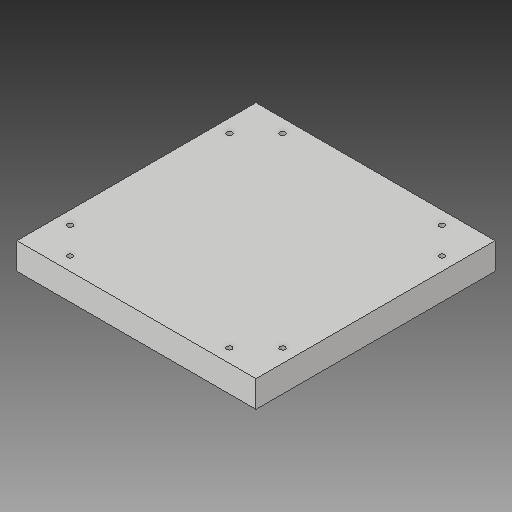
# Autodesk Inventor part: 内层升降板
Saved by Autodesk Inventor 2017 (Build 210142000, 142)
## iProperties
Part Number: 内层升降板
Material: 常规
Document SubType Name: Modeling
Designer: PANDA
Density: 1 g/cm^3
Appearance: 默认
Mass: 645.989 g
Surface Area: 810.096 cm^2
Volume: 645.989 cm^3
Author: PANDA
Autodesk Inventor part; units mm, degrees
ref_plane "YZ Plane" through (0, 0, 0) normal (1, 0, 0) x (0, 1, 0)
ref_plane "XZ Plane" through (0, 0, 0) normal (0, 1, 0) x (-1, 0, 0)
ref_plane "XY Plane" through (0, 0, 0) normal (0, 0, 1) x (1, 0, 0)
sketch "草图2" plane through (0, 0, 0) normal (0, 1, 0) x (-1, 0, 0)
  line L0 (90, 90) -> (-90, 90)
  line L1 (-90, 90) -> (-90, -90)
  line L2 (-90, -90) -> (90, -90)
  line L3 (90, -90) -> (90, 90)
  point P0 (0, 0)
  dimension "d4" = 180
  dimension "d5" = 180
  constraints: 8 end point, 2 parallel, 1 horizontal, 1 perpendicular
  measures "d4" distance of L2.end L1.end
  measures "d5" distance of L1.end L0.end
extrude "拉伸2" add sketch "草图2" along normal blind 20
sketch "草图3" plane through (0, 20, 0) normal (0, 1, 0) x (1, 0, 0)
  circle A0 centre (80, 60) radius 2
  point P0 (0, 0)
  dimension "d8" = 4
  constraints: 1 centre point
  measures "d8" diameter of A0
extrude "拉伸3" cut sketch "草图3" against normal through all
sketch "草图4" plane through (0, 0, 0) normal (0, -1, 0) x (1, 0, 0)
  circle A0 centre (60, -80) radius 2
  point P0 (0, 0)
  dimension "d11" = 4
  constraints: 1 centre point
  measures "d11" diameter of A0
extrude "拉伸4" cut sketch "草图4" against normal through all
sketch "草图5" plane through (0, 0, 0) normal (0, -1, 0) x (1, 0, 0)
  circle A0 centre (80, 60) radius 2
  point P0 (0, 0)
  dimension "d14" = 4
  constraints: 1 centre point
  measures "d14" diameter of A0
extrude "拉伸5" cut sketch "草图5" against normal through all
sketch "草图6" plane through (0, 0, 0) normal (0, -1, 0) x (1, 0, 0)
  circle A0 centre (60, 80) radius 2
  point P0 (0, 0)
  dimension "d17" = 4
  constraints: 1 centre point
  measures "d17" diameter of A0
extrude "拉伸6" cut sketch "草图6" against normal through all
sketch "草图7" plane through (0, 0, 0) normal (0, -1, 0) x (1, 0, 0)
  circle A0 centre (-80, -60) radius 2
  point P0 (0, 0)
  dimension "d20" = 4
  constraints: 1 centre point
  measures "d20" diameter of A0
extrude "拉伸7" cut sketch "草图7" against normal through all
sketch "草图8" plane through (0, 0, 0) normal (0, -1, 0) x (1, 0, 0)
  circle A0 centre (-60, -80) radius 2
  point P0 (0, 0)
  dimension "d23" = 4
  constraints: 1 centre point
  measures "d23" diameter of A0
extrude "拉伸8" cut sketch "草图8" against normal through all
sketch "草图9" plane through (0, 0, 0) normal (0, -1, 0) x (1, 0, 0)
  circle A0 centre (-80, 60) radius 2
  point P0 (0, 0)
  dimension "d26" = 4
  constraints: 1 centre point
  measures "d26" diameter of A0
extrude "拉伸9" cut sketch "草图9" against normal through all
sketch "草图10" plane through (0, 0, 0) normal (0, -1, 0) x (1, 0, 0)
  circle A0 centre (-60, 80) radius 2
  point P0 (0, 0)
  dimension "d29" = 4
  constraints: 1 centre point
  measures "d29" diameter of A0
extrude "拉伸10" cut sketch "草图10" against normal through all
